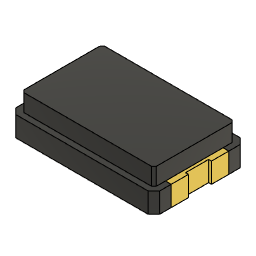
Crystal 2pin 5x3.2mm v1 (Autodesk Fusion 360 design; units mm, degrees)
Autodesk Fusion 360 part; units mm, degrees
sketch "Sketch1" plane through (0, 0, 0) normal (0, 0, 1) x (1, 0, 0)
  line L0 (-2.3, 1.6) -> (2.3, 1.6)
  line L1 (2.3, -1.6) -> (-2.3, -1.6)
  line L2 (-2.5, 1.4) -> (-2.3, 1.6)
  line L3 (2.3, 1.6) -> (2.5, 1.4)
  line L4 (2.5, -1.4) -> (2.3, -1.6)
  line L5 (-2.3, -1.6) -> (-2.5, -1.4)
  line L6 (-2.3, -1.3172) -> (-2.3, 1.3172)
  line L7 (-2.3, 1.3172) -> (-2.2172, 1.4)
  line L8 (-2.2172, 1.4) -> (2.2172, 1.4)
  line L9 (2.2172, 1.4) -> (2.3, 1.3172)
  line L10 (2.3, 1.3172) -> (2.3, -1.3172)
  line L11 (2.3, -1.3172) -> (2.2172, -1.4)
  line L12 (2.2172, -1.4) -> (-2.2172, -1.4)
  line L13 (-2.2172, -1.4) -> (-2.3, -1.3172)
  line L14 (-2.5, 0.4) -> (-2.4, 0.4)
  line L15 (-2.4, 0.4) -> (-2.4, -0.4)
  line L16 (-2.4, -0.4) -> (-2.5, -0.4)
  line L17 (2.5, 0.4) -> (2.4, 0.4)
  line L18 (2.4, 0.4) -> (2.4, -0.4)
  line L19 (2.4, -0.4) -> (2.5, -0.4)
  line L20 (-2.5, -1.4) -> (-2.5, -0.4)
  line L21 (-2.5, 0.4) -> (-2.5, 1.4)
  line L22 (2.5, 1.4) -> (2.5, 0.4)
  line L23 (2.5, -0.4) -> (2.5, -1.4)
  line L24 (2.5, -1) -> (2.3, -1)
  line L25 (-2.3, -1) -> (-2.5, -1)
  line L26 (-2.5, 1) -> (-2.3, 1)
  line L27 (2.3, 1) -> (2.5, 1)
  line L28 (-2.3, -1) -> (-1.2, -1)
  line L29 (-1.2, -1) -> (-1.2, 1)
  line L30 (-1.2, 1) -> (-2.3, 1)
  line L31 (2.3, -1) -> (1.2, -1)
  line L32 (1.2, -1) -> (1.2, 1)
  line L33 (1.2, 1) -> (2.3, 1)
  constraint horizontal L0
  constraint vertical L22
  constraint horizontal L1
  constraint vertical L20
  constraint perpendicular L2 L3
  constraint perpendicular L4 L5
  constraint horizontal L14
  constraint vertical L15
  constraint horizontal L16
  constraint horizontal L17
  constraint vertical L18
  constraint horizontal L19
  constraint coincident L14.start L20
  constraint collinear L20 L21
  constraint coincident L19.end L22
  constraint collinear L22 L23
  constraint horizontal L26
  constraint horizontal L24
  constraint coincident L21 L26.start
  constraint coincident L20 L25.end
  constraint coincident L23 L24.start
  constraint coincident L22 L27.end
  constraint coincident L10 L24.end
  constraint coincident L6 L25.start
  constraint collinear L24 L25
  constraint coincident L6 L26.end
  constraint coincident L10 L27.start
  constraint collinear L26 L27
  constraint perpendicular L10 L28
  constraint perpendicular L28 L29
  constraint perpendicular L29 L30
  constraint perpendicular L10 L31
  constraint perpendicular L31 L32
  constraint perpendicular L32 L33
extrude "Extrude2" add sketch "Sketch1" along normal blind 0.6 contours L6 L28 L29 L30 | L6 L7 L8 L9 L10 L11 L12 L13 L28 L29 L30 L31 L32 L33 | L10 L31 L32 L33 makes body 1
extrude "Extrude1" add sketch "Sketch1" along normal blind 0.7 separate body makes body 2
move_body "Move1" bodies 1 to x (1, 0, 0) y (0, 1, 0) z (0, 0, 1) at (0, 0, 0.7)
extrude "Extrude3" add sketch "Sketch1" along normal blind 0.2 separate body contours L6 L28 L29 L30 | L10 L31 L32 L33 makes body 3 at (-1.9333, 0.3333, 0) makes body 4 at (1.9333, -0.3333, 0)
extrude "Extrude4" add sketch "Sketch1" along normal blind 0.7 contours L6 L14 L15 L16 L20 L21 L25 L26 | L10 L17 L18 L19 L22 L23 L24 L27 bodies 3 4
extrude "Extrude5" cut sketch "Sketch1" along normal blind 0.9 contours L10 L17 L18 L19 L22 L23 L24 L27 bodies 2
extrude "Extrude6" cut sketch "Sketch1" along normal blind 1.1 contours L6 L14 L15 L16 L20 L21 L25 L26 bodies 2
extrude "Extrude7" cut sketch "Sketch1" along normal blind 0.2 contours L6 L28 L29 L30 | L10 L31 L32 L33 bodies 2
